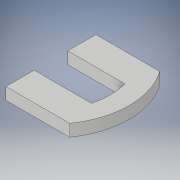
# Autodesk Inventor part: BUTTON_TOP
Saved by Autodesk Inventor 2019 (Build 230136000, 136)
## iProperties
Created: 2018-12-19
Part Number: BUTTON_TOP
Material: Типовые
Document SubType Name: Modeling
Designer: aldanstar
Density: 1 g/cm^3
Appearance: По умолчанию
Author: aldanstar
Autodesk Inventor part; units mm, degrees
ref_plane "YZ Plane" through (0, 0, 0) normal (1, 0, 0) x (0, 1, 0)
ref_plane "XZ Plane" through (0, 0, 0) normal (0, 1, 0) x (-1, 0, 0)
ref_plane "XY Plane" through (0, 0, 0) normal (0, 0, 1) x (1, 0, 0)
sketch "Эскиз1" plane through (0, 0, 0) normal (0, 1, 0) x (-1, 0, 0)
  line L0 (2.6545, 3.75) -> (-2.6545, 3.75)
  line L1 (-2.6545, 3.75) -> (-2.6545, -3.75) construction
  line L2 (-2.6545, -3.75) -> (2.6545, -3.75)
  line L3 (2.6545, -3.75) -> (2.6545, 3.75)
  line L4 (3.9547, 0) -> (-5.1453, 0) projected
  line L5 (0, -5.25) -> (0, 5.25) projected
  arc A0 (-2.6545, 3.75) -> (-2.6545, -3.75) centre (2.6547, 0) ccw
  point P0 (0, 0)
  dimension "d0" = 5.309
  dimension "d1" = 7.5
  dimension "d2" = 6.5
  constraints: 8 end point, 2 parallel, 2 point on circle, 1 centre point, 1 horizontal, 1 perpendicular, 2 other
  measures "d0" distance of L1.end L2.end
  measures "d1" distance of L2.end L0.start
  measures "d2" radius of A0
extrude "Выдавливание1" add sketch "Эскиз1" along normal blind 1
sketch "Эскиз2" plane through (0, 1, 0) normal (0, 1, 0) x (1, 0, 0)
  line L0 (-2.6545, 3.75) -> (-2.6545, -3.75) projected
  line L1 (-2.6545, -1.4) -> (2.1155, -1.4)
  line L2 (2.1155, -1.4) -> (2.1155, 1.4) construction
  line L3 (2.1155, 1.4) -> (-2.6545, 1.4)
  line L4 (-2.6545, 1.4) -> (-2.6545, -1.4)
  line L5 (-4.6131, 0) -> (5.255, 0) projected
  arc A0 (2.1155, -1.4) -> (2.1155, 1.4) centre (-3.2033, 0) ccw
  point P0 (0, 0)
  dimension "d5" = 4.77
  dimension "d6" = 2.8
  dimension "d7" = 5.5
  constraints: 8 end point, 2 parallel, 2 point on circle, 1 centre point, 1 horizontal, 1 perpendicular, 1 point on line, 1 other
  measures "d5" distance of L2.end L3.end
  measures "d6" distance of L1.end L2.end
  measures "d7" radius of A0
extrude "Выдавливание2" cut sketch "Эскиз2" against normal through all
